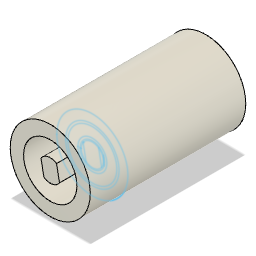
proto2 v6 (Autodesk Fusion 360 design; units mm, degrees)
Autodesk Fusion 360 part; units mm, degrees
note: some values were not read from the file. Chosen so that the rebuilt part matches the saved one: which bodies a step acts on; which face or edge a step refers to. Set by a fixed rule: which sketch regions a step uses.
sketch "Esquisse1" plane through (0, 0, 0) normal (0, 0, 1) x (1, 0, 0)
  circle A0 centre (40.0644, 42.4514) radius 40
  circle A1 centre (40.0644, 42.4514) radius 7
  circle A2 centre (40.0644, 42.4514) radius 30
  line L0 (40.1722, 49.4505) -> (40.1722, 72.4512)
  line L1 (37.8965, 49.1072) -> (32.2094, 71.4048)
  line L2 (46.7763, 71.6909) -> (42.0309, 49.1695)
  line L3 (33.0644, 42.4463) -> (10.1007, 43.928)
  line L4 (14.33, 57.8703) -> (34.2828, 46.3976)
  line L5 (37.906, 35.7924) -> (29.4008, 14.4105)
  line L6 (17.4477, 22.7413) -> (34.5246, 38.1722)
  line L7 (45.7304, 38.3409) -> (63.4375, 23.6446)
  line L8 (51.8209, 14.8509) -> (42.4222, 35.8604)
  line L9 (45.7245, 46.5699) -> (65.1734, 58.8689)
  line L10 (69.9469, 45.1034) -> (47.0613, 42.6571)
  circle A3 centre (40.0644, 42.4514) radius 1
  dimension "d1" = 80
  dimension "d2" = 14
  dimension "d3" = 60
  dimension "d5" = 360
  dimension "d8" = 2
  constraint concentric A0 A1
  constraint concentric A0 A2
  constraint coincident A1 L0.start
  constraint coincident A2 L0.end
  constraint vertical L0
  constraint coincident A1 L1.start
  constraint coincident A2 L1.end
  constraint coincident A2 L2.start
  constraint coincident A1 L2.end
  constraint concentric A2 A3
  measures "d1" diameter of A0
  measures "d2" diameter of A1
  measures "d3" diameter of A2
  measures "d8" diameter of A3
combine "Combiner1" [no effect]
sketch "Esquisse2" plane through (0, 0, 0) normal (1, 0, 0) x (0, 0, -1)
  line L0 (-137, 50) -> (-137, 7)
  constraint vertical L0
sketch "Esquisse3" plane through (0, 50, 0) normal (0, 1, 0) x (-1, 0, 0)
  line L0 (-40, 137) -> (0, 137)
ref_plane "Plan de construction1" through (20, 28.5, 137) normal (0, 0, -1) x (0, 1, 0)
sketch "Esquisse5" plane through (20, 28.5, 137) normal (0, 0, -1) x (1, 0, 0)
  line L0 (20, 21.5) -> (-20, -21.5) construction
sketch "Esquisse6" plane through (0, 0, 137) normal (0, 0, -1) x (-1, 0, 0)
  line L0 (0, 7) -> (0, 50)
  line L1 (0, 50) -> (-40, 50)
  line L2 (-40, 50) -> (-40, 7)
  line L3 (-40, 7) -> (0, 7)
  line L4 (-40, 7) -> (0, 50) construction
  circle A0 centre (-20, 28.5) radius 12.5
  circle A1 centre (-20, 28.5) radius 5
  circle A2 centre (-20, 28.5) radius 2.5
  line L5 (-40, 50) -> (3, 50)
  line L6 (3, 50) -> (3, 7)
  line L7 (3, 7) -> (-40, 7)
  line L8 (-40, 7) -> (-40, 50)
  dimension "d48" = 25
  dimension "d49" = 10
  dimension "d50" = 5
  dimension "d55" = 43
  constraint coincident L2.end L3.start
  constraint coincident L0.end L1.start
  constraint midpoint L4 A0.centre
  constraint concentric A0 A1
  constraint concentric A1 A2
  constraint horizontal L5
  constraint vertical L6
  constraint horizontal L7
  constraint vertical L8
  constraint coincident L1.end L2.start
  measures "d48" diameter of A0
  measures "d49" diameter of A1
  measures "d50" diameter of A2
  measures "d55" distance of L1.end L5.end
combine "Combiner2" [no effect]
sketch "Esquisse7" plane through (0, 0, 0) normal (0, 1, 0) x (1, 0, 0)
sketch "Esquisse8" plane through (0, 0, 112) normal (0, 0, -1) x (-1, 0, 0)
  circle A0 centre (-20, 28.5) radius 2.5
  circle A1 centre (-20, 28.5) radius 2.5
  circle A2 centre (-20, 28.5) radius 2.75
  circle A3 centre (-20, 28.5) radius 3.25
  line L0 (-17.9875, 29.9832) -> (-18.1, 29.9832)
  line L1 (-17.9129, 29.8763) -> (-18.5823, 26.4409)
  line L2 (-22.0871, 27.1237) -> (-21.4177, 30.5591)
  line L3 (-22.6153, 27.65) -> (-22.4995, 29.6467)
  circle A4 centre (-20, 28.5) radius 5.5
  circle A5 centre (-20, 28.5) radius 8
  circle A6 centre (-20, 28.5) radius 6
  dimension "d93" = 5
  dimension "d122" = 5.5
  dimension "d123" = 6.5
  dimension "d124" = 3.5
  dimension "d127" = 2
  dimension "d136" = 11
  dimension "d145" = 16
  dimension "d158" = 12
  constraint concentric A1 A2
  constraint coincident A1 L0.start
  constraint horizontal L0
  constraint coincident A1 L1.start
  constraint coincident A1 L1.end
  constraint coincident A2 L3.start
  constraint coincident A2 L3.end
  constraint concentric A3 A4
  constraint concentric A4 A5
  constraint concentric A5 A6
  measures "d93" diameter of A1
  measures "d122" diameter of A2
  measures "d123" diameter of A3
  measures "d124" distance of L1.start L1.end
  measures "d127" distance of L3.start L3.end
  measures "d136" diameter of A4
  measures "d145" diameter of A5
  measures "d158" diameter of A6
extrude "Extrusion34" add sketch "Esquisse8" along normal blind 20 contours A2 L3 | A3 picked at (-22.5856, 28.8533) makes body 1
extrude "Extrusion29" add sketch "Esquisse8" along normal blind 25 separate body contours A0 A1 L1 | A0 A1 L1 L2 | A0 A1 L2 makes body 2
extrude "Extrusion30" add sketch "Esquisse8" along normal blind 3 contours A0 A1 L1 | A0 A1 L2 bodies 2
extrude "Extrusion31" add sketch "Esquisse8" against normal blind 30 contours A0 A1 L1 | A0 A1 L1 L2 | A0 A1 L2 bodies 2
move_body "Déplacer9" bodies 2 to x (1, 0, 0) y (0, 1, 0) z (0, 0, 1) at (66, 0, 0)
extrude "Extrusion32" cut 1 faces at (87.1935, 29.0835, 142) along direction (0, 0, -1) blind 5 on bodies 2 bodies 2
extrude "Extrusion33" cut 1 faces at (85.3115, 28.9694, 87) along direction (0, 0, 1) blind 10 on bodies 2 bodies 2
sketch "Esquisse9" plane through (7.6522, -14.5112, 0) normal (0.466451, -0.884547, 0) x (0, 0, -1)
  line L0 (-97, 87.3649) -> (-97, 91.3649)
  line L1 (-97, 91.3649) -> (-109, 91.3649)
  line L2 (-417.5, 94.5) -> (-401.9765, 92.2725)
  line L3 (-401.9765, 92.2725) -> (-415, 97.5)
  line L4 (-109, 91.3649) -> (-112, 91.3649)
  line L5 (-112, 91.3649) -> (-112, 87.3649)
  line L6 (-112, 87.3649) -> (-109, 87.3649)
  line L7 (-109, 87.3649) -> (-97, 87.3649)
ref_plane "Plan de construction3" through (20, 28.5, 112) normal (0, 0, -1) x (-1, 0, 0)
extrude "Extrusion35" add sketch "Esquisse8" against normal blind 10 separate body contours A0 A1 L1 L2 makes body 3
extrude "Extrusion36" add sketch "Esquisse8" against normal blind 3 contours A0 A1 L2 | A2 L3 | A2 L3 | A3 bodies 1 3
extrude "Extrusion37" add sketch "Esquisse8" against normal blind 3 contours A0 A1 L1 bodies 1
copy_body "Corps->Comp5" bodies 1 removing the originals makes body 4 in component "axe4"
extrude "Extrusion1" add sketch "Esquisse8" against normal blind 9.5 contours A4 bodies 4 in component "axe4"
extrude "Extrusion2" add 1 faces at (15.2705, 28.2268, 112) along direction (0, 0, -1) blind 2 on bodies 4 bodies 4 in component "axe4"
extrude "Extrusion3" add 1 faces at (15.2705, 28.2268, 110) along direction (0, 0, -1) blind 2.5 on bodies 4 bodies 4 in component "axe4"
extrude "Extrusion4" cut 1 faces at (15.2705, 28.2268, 121.5) along direction (0, 0, -1) blind 14 on bodies 4 bodies 4 in component "axe4"
extrude "Extrusion38" add sketch "Esquisse8" against normal blind 10 separate body contours A5 | A6 makes body 5
extrude "Extrusion39" add sketch "Esquisse8" along normal blind 5 contours A4 | A5 | A6 bodies 5
extrude "Extrusion40" add sketch "Esquisse8" against normal blind 1 contours A4 bodies 5
extrude "Extrusion41" add 1 faces at (15.2705, 28.2268, 113) along direction (0, 0, 1) blind 2 on bodies 5 bodies 5
copy_body "Corps->Comp6" bodies 5 removing the originals makes body 6 in component "Component"
copy_body "CutPasteBodies1" bodies 6 removing the originals makes body 7 in component "axe4"
extrude "Extrusion5" cut 1 faces at (12.8836, 27.8293, 122) along direction (0, 0, -1) blind 10 on bodies 7 bodies 7 in component "axe4"
extrude "Extrusion6" cut 2 faces at (15.2705, 28.2268, 115) (22.2395, 28.8891, 115) along direction (0, 0, -1) blind 3 on bodies 4 7 bodies 4 7 makes body 8 at (16.7661, 28.8236, 105.3333) in component "axe4"
extrude "Extrusion7" add sketch "Esquisse8" against normal blind 10 contours A5 bodies 7 in component "axe4"
extrude "Extrusion8" add sketch "Esquisse8" along normal blind 3 contours A0 A1 L1 | A2 L3 | A2 L3 bodies 8 4 in component "axe4"
extrude "Extrusion9" add sketch "Esquisse8" along normal blind 3 contours A0 A1 L1 L2 | A0 A1 L2 bodies 8 in component "axe4"
extrude "Extrusion10" add 1 faces at (18.2601, 27.9948, 109) along direction (0, 0, -1) blind 3 on bodies 8 bodies 8 in component "axe4"
sketch "Esquisse10" plane through (0, 0, 107) normal (0, 0, -1) x (-1, 0, 0)
  circle A0 centre (-20, 28.5) radius 3.25
  circle A1 centre (-20, 28.5) radius 8
  circle A2 centre (-20, 28.5) radius 6.5251
  line L0 (0, 36.5) -> (0, 38.5)
  constraint concentric A0 A2
  constraint vertical L0
ref_plane "Plan de construction5" through (20, 28.5, 103) normal (0, 0, -1) x (-1, 0, 0)
sketch "Esquisse11" plane through (20, 28.5, 103) normal (0, 0, -1) x (1, 0, 0)
  line L0 (0, -8) -> (0, 8) construction
  circle A0 centre (0, 0) radius 3.2504
  constraint vertical L0
  constraint coincident A0.centre origin
loft "Lissage1" add profiles "Esquisse11", "Esquisse10" section 1 section 2 contours A1 bodies 8 7 in component "axe4"
delete_face "DeleteFace1" 1 faces at (21.5453, 35.2704, 106.1111) on bodies 8 in component "axe4"
extrude "Extrusion11" add 1 faces at (13.6252, 27.9411, 103) along direction (0, 0, -1) blind 11 on bodies 8 bodies 8 in component "axe4"
extrude "Extrusion12" add 2 faces at (13.6252, 27.9411, 92) (22.7883, 28.5989, 92) along direction (0, 0, -1) blind 5 on bodies 8 bodies 8 in component "axe4"
move_face "DécalerLesFaces1" offset 1 3 faces at (12.0099, 28.1012, 88.6667) (12.0099, 28.1012, 95.6667) (12.0099, 28.1012, 115.6667) on bodies 8 in component "axe4"
component "axe4" placed x (1, 0, 0) y (0, 1, 0) z (0, 0, 1) at (0, 0, 0)
component "Component" placed x (1, 0, 0) y (0, 1, 0) z (0, 0, 1) at (0, 0, 0) in component "axe4"
hidden bodies 2
named bodies: "axe2"
